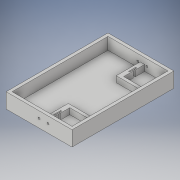
# Autodesk Inventor part: P1794_001_basManette
Saved by Autodesk Inventor 2019 (Build 230136000, 136)
## iProperties
Created: 2019-04-29
Part Number: P1794_001_basManette
Material: Générique
Document SubType Name: Modeling
Designer: Joan.MAILLARD
Density: 1 g/cm^3
Appearance: Par défaut
Author: Joan.MAILLARD
Autodesk Inventor part; units mm, degrees
ref_plane "YZ Plane" through (0, 0, 0) normal (1, 0, 0) x (0, 1, 0)
ref_plane "XZ Plane" through (0, 0, 0) normal (0, 1, 0) x (-1, 0, 0)
ref_plane "XY Plane" through (0, 0, 0) normal (0, 0, 1) x (1, 0, 0)
sketch "Esquisse1" plane through (0, 0, 0) normal (0, 1, 0) x (-1, 0, 0)
  line L0 (-55, 85) -> (55, 85)
  line L1 (55, 85) -> (55, -85)
  line L2 (55, -85) -> (-55, -85)
  line L3 (-55, -85) -> (-55, 85)
  line L4 (-55, 85) -> (55, -85) construction
  line L5 (55, 85) -> (-55, -85) construction
  point P0 (0, 0)
  dimension "d0" = 170
  dimension "d1" = 110
  constraints: 12 end point, 2 midpoint, 2 parallel, 1 horizontal, 1 perpendicular
  measures "d0" distance of L0.end L1.end
  measures "d1" distance of L1.end L2.end
extrude "Extrusion1" add sketch "Esquisse1" along normal blind 25
sketch "Esquisse2" plane through (0, 25, 0) normal (0, 1, 0) x (1, 0, 0)
  line L0 (-50, -80) -> (50, -80)
  line L1 (50, -80) -> (50, 80)
  line L2 (50, 80) -> (-50, 80)
  line L3 (-50, 80) -> (-50, -80)
  line L4 (-50, -80) -> (50, 80) construction
  line L5 (50, -80) -> (-50, 80) construction
  line L6 (55, 85) -> (-55, 85) projected
  line L7 (-55, 85) -> (-55, -85) projected
  point P0 (0, 0)
  dimension "d66" = 5
  dimension "d67" = 5
  constraints: 12 end point, 2 midpoint, 2 parallel, 1 horizontal, 1 perpendicular
  measures "d66" distance between parallel lines of L6 L2
  measures "d67" distance between parallel lines of L7 L3
extrude "Extrusion2" cut sketch "Esquisse2" against normal blind 20
sketch "Esquisse3" plane through (55, 0, -85) normal (0, 0, -1) x (-1, 0, 0)
  line L0 (55, 14) -> (40, 14) construction
  line L1 (110, 0) -> (0, 0) construction
  line L2 (0, 0) -> (0, 25) construction
  point P0 (55, 0)
  point P1 (105, 0)
  point P2 (0, 20)
  dimension "d15" = 14
  dimension "d16" = 15
  dimension "d17" = 40
  constraints: 2 end point, 1 horizontal
  measures "d15" distance between parallel lines of L1 L0
  measures "d16" distance of L0.end L0.start
  measures "d17" distance from line of L2 L0.end
hole "Perçage1" at (15, 14, -85) at (0, 14, -85) direction (0, 0, 1) diameter 3.4 depth 8.8 tip angle 118 clearance for "Vis à tête plate fraisée ISO 2009/7046" size "M3" standard "ISO"
sketch "Esquisse6" plane through (0, 5, 0) normal (0, 1, 0) x (1, 0, 0)
  line L0 (50, 45) -> (11.25, 45)
  line L1 (11.25, 45) -> (11.25, 40)
  line L2 (11.25, 40) -> (50, 40)
  line L3 (50, 40) -> (50, 45)
  line L4 (11.25, 40) -> (3.75, 40)
  line L5 (3.75, 40) -> (3.75, 80)
  line L6 (3.75, 80) -> (11.25, 80)
  line L7 (11.25, 80) -> (11.25, 40)
  line L8 (11.25, -80) -> (3.75, -80)
  line L9 (3.75, -80) -> (3.75, -40)
  line L10 (3.75, -40) -> (11.25, -40)
  line L11 (11.25, -40) -> (11.25, -80)
  line L12 (50, -40) -> (11.25, -40)
  line L13 (11.25, -40) -> (11.25, -45)
  line L14 (11.25, -45) -> (50, -45)
  line L15 (50, -45) -> (50, -40)
  line L16 (-50, 80) -> (50, 80) projected
  line L17 (50, 80) -> (50, -80) projected
  line L18 (50, -80) -> (-50, -80) projected
  point P0 (0, 0)
  point P1 (7.5, -40)
  dimension "d44" = 5
  dimension "d45" = 7.5
  dimension "d48" = 5
  dimension "d50" = 7.5
  dimension "d70" = 35
  dimension "d71" = 38.75
  dimension "d72" = 38.75
  dimension "d73" = 35
  constraints: 32 end point, 8 parallel, 6 point on line, 4 horizontal, 4 perpendicular, 1 midpoint
  measures "d44" distance between parallel lines of L2 L0
  measures "d45" distance between parallel lines of L5 L7
  measures "d48" distance between parallel lines of L14 L12
  measures "d50" distance between parallel lines of L11 L9
  measures "d70" distance between parallel lines of L0 L16
  measures "d71" distance between parallel lines of L17 L11
  measures "d72" distance between parallel lines of L17 L7
  measures "d73" distance between parallel lines of L18 L14
extrude "Extrusion4" add sketch "Esquisse6" along normal blind 10 contours L3 L2 L1 L0 | L1 L4 L5 L6 L7 | L8 L9 L10 L11 | L11 L12 L15 L14
sketch "Esquisse9" plane through (0, 15, 0) normal (0, 1, 0) x (1, 0, 0)
  line L0 (7.75, 68.5) -> (9.75, 68.5)
  line L1 (9.75, 68.5) -> (9.75, 56.5)
  line L2 (9.75, 56.5) -> (7.75, 56.5)
  line L3 (7.75, 56.5) -> (7.75, 68.5)
  line L4 (7.75, -56.5) -> (9.75, -56.5)
  line L5 (9.75, -56.5) -> (9.75, -68.5)
  line L6 (9.75, -68.5) -> (7.75, -68.5)
  line L7 (7.75, -68.5) -> (7.75, -56.5)
  line L8 (11.25, 80) -> (11.25, 45) projected
  line L9 (9.75, 64) -> (11.25, 64)
  line L10 (11.25, 64) -> (11.25, 61)
  line L11 (11.25, 61) -> (9.75, 61)
  line L12 (9.75, 61) -> (9.75, 64)
  line L13 (11.25, -45) -> (11.25, -80) projected
  line L14 (9.75, 68.5) -> (11.25, 64) construction
  line L15 (9.75, 56.5) -> (11.25, 61) construction
  line L16 (8.75, 68.5) -> (8.75, 80) construction
  line L17 (11.25, 45) -> (3.75, 45) construction
  line L18 (3.75, 80) -> (3.75, 40) construction
  line L19 (8.75, 56.5) -> (8.75, 45) construction
  line L20 (-50, 80) -> (50, 80) construction
  line L21 (11.25, -45) -> (3.75, -45) construction
  line L22 (3.75, -80) -> (3.75, -40) construction
  line L23 (8.75, -56.5) -> (8.75, -45) construction
  line L24 (8.75, -68.5) -> (8.75, -80) construction
  line L25 (50, -80) -> (-50, -80) construction
  line L26 (9.75, -64) -> (11.25, -64)
  line L27 (11.25, -64) -> (11.25, -61)
  line L28 (11.25, -61) -> (9.75, -61)
  line L29 (9.75, -61) -> (9.75, -64)
  line L30 (11.25, -61) -> (9.75, -56.5) construction
  line L31 (11.25, -64) -> (9.75, -68.5) construction
  point P0 (0, 0)
  dimension "d74" = 12
  dimension "d75" = 3
  dimension "d78" = 2
  dimension "d79" = 4
  dimension "d80" = 12
  dimension "d82" = 3
  constraints: 52 end point, 13 point on line, 8 parallel, 6 horizontal, 6 perpendicular, 4 equal length, 4 midpoint, 1 vertical
  measures "d74" distance between parallel lines of L2 L0
  measures "d75" distance between parallel lines of L11 L9
  measures "d78" distance between parallel lines of L12 L3
  measures "d79" distance between parallel lines of L3 L18
  measures "d80" distance of L6.end L4.start
  measures "d82" distance between parallel lines of L26 L28
extrude "Extrusion5" cut sketch "Esquisse9" against normal blind 10
sketch "Esquisse10" plane through (-55, 0, 85) normal (0, 0, 1) x (1, 0, 0)
  point P0 (55, 0)
  point P1 (55, 14)
  point P2 (70, 14)
  point P3 (70, 14)
  point P4 (55, 14)
  constraints: 2 coincident
hole "Perçage5" at (0, 14, 85) at (15, 14, 85) direction (0, 0, -1) diameter 3.4 depth 8.8 tip angle 118 clearance for "Vis à tête plate fraisée ISO 2009/7046" size "M3" standard "ISO"
equation "\"d67\" = d66"
equation "\"d45\" = 1.5 * d44"
equation "\"d50\" = d45"
equation "\"d72\" = d71"
equation "\"d73\" = d70"
equation "\"d80\" = d74"
equation "\"d82\" = d75"
